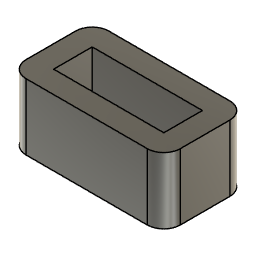
ballzbarbumber v3 (Autodesk Fusion 360 design; units mm, degrees)
Autodesk Fusion 360 part; units mm, degrees
sketch "Sketch1" plane through (0, 0, 0) normal (0, 0, 1) x (1, 0, 0)
  line L0 (5, 1.75) -> (-5, 1.75)
  line L1 (-5, 1.75) -> (-5, -1.75)
  line L2 (-5, -1.75) -> (5, -1.75)
  line L3 (5, -1.75) -> (5, 1.75)
  line L4 (5, 1.75) -> (-5, -1.75) construction
  line L5 (-5, 1.75) -> (5, -1.75) construction
  line L6 (-7, -3.75) -> (7, -3.75)
  line L7 (7, -3.75) -> (7, 3.75)
  line L8 (7, 3.75) -> (-7, 3.75)
  line L9 (-7, 3.75) -> (-7, -3.75)
  dimension "d1" = 10
  dimension "d2" = 3.5
  dimension "d3" = 2
  constraint horizontal L0
  constraint perpendicular L0 L1
  constraint parallel L0 L2
  constraint parallel L1 L3
  constraint coincident L4 origin
  constraint coincident L5 origin
  measures "d1" distance of L1.end L2.end
  measures "d2" distance of L0.end L1.end
extrude "Extrude1" add sketch "Sketch1" along normal blind 6
fillet "Fillet2" radius 1.5 4 edges at (7, 3.75, 3) (-7, 3.75, 3) (-7, -3.75, 3) (7, -3.75, 3)
